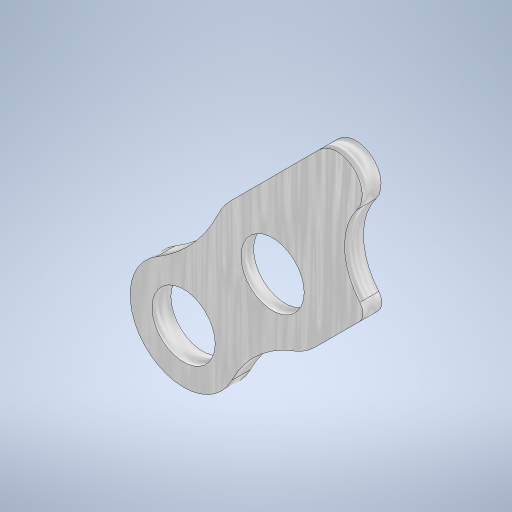
# Autodesk Inventor part: dsa
Saved by Autodesk Inventor 2023 (Build 270158000, 158)
## iProperties
Created: 2022-04-10
Part Number: dsa
Material: Aluminum 7075
Document SubType Name: Modeling
Designer: acps
Density: 2.81 g/cm^3
Appearance: Satin - Brushed Heavy
Author: acps
Autodesk Inventor part; units mm, degrees
ref_plane "YZ Plane" through (0, 0, 0) normal (1, 0, 0) x (0, 1, 0)
ref_plane "XZ Plane" through (0, 0, 0) normal (0, 1, 0) x (-1, 0, 0)
ref_plane "XY Plane" through (0, 0, 0) normal (0, 0, 1) x (1, 0, 0)
sketch "Sketch1" plane through (0, 0, 0) normal (0, 0, 1) x (1, 0, 0)
  circle A0 centre (47, 53.101) radius 5.025
  line L0 (47, 53.101) -> (61.1421, 67.2432) construction
  circle A1 centre (61.1421, 67.2432) radius 5.025
  circle A2 centre (61.1421, 67.2432) radius 9.5
  circle A3 centre (47, 53.101) radius 8.5
  line L1 (68.5668, 88.1028) -> (54.4246, 73.9607)
  arc A4 (74.5933, 82.8719) -> (68.5668, 88.1028) centre (71.3952, 85.2744) ccw
  arc A5 (74.5933, 82.8719) -> (75.0285, 70.3201) centre (82.5886, 76.8657) ccw
  arc A6 (74.9307, 67.5967) -> (75.0285, 70.3201) centre (73.5165, 69.0109) ccw
  line L2 (74.9307, 67.5967) -> (67.8597, 60.5257)
  circle A7 centre (47, 53.101) radius 7.5
  circle A8 centre (61.1421, 67.2432) radius 7.5
  arc A9 (42.6661, 60.4132) -> (52.5446, 71.2845) centre (29.9195, 81.9195) ccw
  arc A10 (64.4883, 58.352) -> (54.6431, 49.3817) centre (70.8284, 41.5055) ccw
  line L3 (124.9643, 38.1784) -> (101.7414, 38.1784) construction
  point P0 (0, 0)
  dimension "d33" = 10.05
  dimension "d34" = 20
  dimension "d35" = 10.05
  dimension "d36" = 19
  dimension "d37" = 17
  dimension "d38" = 4
  dimension "d39" = 2
  dimension "d40" = 10
  dimension "d41" = 20
  dimension "d42" = 10
  dimension "d43" = 15
  dimension "d44" = 15
  dimension "d45" = 25
  dimension "d46" = 18
  dimension "d47" = 45
  constraints: 16 point on circle, 11 centre point, 10 tangent, 8 end point, 6 coincident, 2 parallel, 1 horizontal, 1 other
  measures "d33" diameter of A0
  measures "d34" distance of L0.start L0.end
  measures "d35" diameter of A1
  measures "d36" diameter of A2
  measures "d37" diameter of A3
  measures "d38" radius of A4
  measures "d39" radius of A6
  measures "d40" radius of A5
  measures "d41" distance of L1.start L1.end
  measures "d42" distance of L2.start L2.end
  measures "d43" diameter of A7
  measures "d44" diameter of A8
  measures "d45" radius of A9
  measures "d46" radius of A10
  measures "d47" angle of L3 L0
extrude "Extrusion1" add sketch "Sketch1" against normal blind 3 contours A2 | A2 L1 A4 A5 A6 L2 | A2 A10 A3 A9 | A3 | A7
extrude "Extrusion2" add sketch "Sketch1" against normal blind 2 contours A8
body "Solid1"
